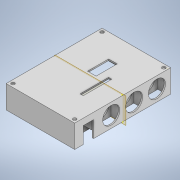
# Autodesk Inventor part: upper casing
Saved by Autodesk Inventor 2020 (Build 240168000, 168)
## iProperties
Created: 2019-06-23
Part Number: upper casing
Material: Generic
Document SubType Name: Modeling
Designer: jjsch
Density: 1 g/cm^3
Appearance: Default
Mass: 122.715 g
Surface Area: 805.458 cm^2
Volume: 122.715 cm^3
Author: jjsch
Autodesk Inventor part; units mm, degrees
ref_plane "YZ Plane" through (0, 0, 0) normal (1, 0, 0) x (0, 1, 0)
ref_plane "XZ Plane" through (0, 0, 0) normal (0, 1, 0) x (-1, 0, 0)
ref_plane "XY Plane" through (0, 0, 0) normal (0, 0, 1) x (1, 0, 0)
sketch "Sketch1" plane through (0, 0, 0) normal (0, 1, 0) x (-1, 0, 0)
  line L0 (-1.2, -80) -> (1.2, -80)
  line L1 (1.2, -80) -> (1.2, 80)
  line L2 (1.2, 80) -> (-1.2, 80)
  line L3 (-1.2, 80) -> (-1.2, -80)
  line L4 (-1.2, -80) -> (1.2, 80) construction
  line L5 (1.2, -80) -> (-1.2, 80) construction
  point P0 (0, 0)
  dimension "d0" = 2.4
  dimension "d1" = 160
  constraints: 12 end point, 2 midpoint, 2 parallel, 1 horizontal, 1 perpendicular
  measures "d0" distance of L2.end L1.end
  measures "d1" distance of L1.end L0.end
extrude "Extrusion1" add sketch "Sketch1" along normal blind 40
sketch "Sketch2" plane through (1.2, 0, 80) normal (1, 0, 0) x (0, 0, -1)
  line L0 (0, 0) -> (0, 40) projected
  line L1 (160, 0) -> (160, 40) projected
  circle A0 centre (60, 20) radius 15
  circle A1 centre (100, 20) radius 15
  circle A2 centre (140, 20) radius 15
  line L2 (29.05, 28.75) -> (10.95, 28.75)
  line L3 (10.95, 28.75) -> (10.95, 11.25)
  line L4 (10.95, 11.25) -> (29.05, 11.25)
  line L5 (29.05, 11.25) -> (29.05, 28.75)
  line L6 (29.05, 28.75) -> (10.95, 11.25) construction
  line L7 (10.95, 28.75) -> (29.05, 11.25) construction
  point P0 (80, 0)
  point P1 (20, 20)
  dimension "d4" = 60
  dimension "d5" = 20
  dimension "d6" = 40
  dimension "d7" = 20
  dimension "d8" = 30
  dimension "d9" = 30
  dimension "d10" = 30
  dimension "d11" = 18.1
  dimension "d12" = 17.5
  constraints: 12 end point, 3 centre point, 3 coincident, 2 midpoint, 2 parallel, 1 horizontal, 1 perpendicular
  measures "d4" distance from line of L0 point (60, 20)
  measures "d5" distance from line of L1 point (140, 20)
  measures "d6" distance of point (140, 20) point (100, 20)
  measures "d7" distance from line of L0 point (20, 20)
  measures "d8" diameter of A0
  measures "d9" diameter of A1
  measures "d10" diameter of A2
  measures "d11" distance of L4.end L3.end
  measures "d12" distance of L3.end L2.end
extrude "Extrusion2" cut sketch "Sketch2" against normal blind 40
sketch "Sketch3" plane through (1.2, 0, -80) normal (0, 0, -1) x (-1, 0, 0)
  line L0 (2.4, 0) -> (2.4, 40) projected
  point P0 (1.2, 0)
sketch "Sketch4" plane through (0, 40, 0) normal (0, 1, 0) x (1, 0, 0)
  line L0 (1.2, -80) -> (-118.8, -80)
  line L1 (-118.8, -80) -> (-118.8, 80)
  line L2 (-118.8, 80) -> (1.2, 80)
  line L3 (1.2, 80) -> (1.2, -80)
  point P0 (0, 0)
  dimension "d17" = 120
  dimension "d18" = 160
  constraints: 8 end point, 2 parallel, 1 horizontal, 1 perpendicular
  measures "d17" distance of L1.end L2.end
  measures "d18" distance of L0.end L1.end
extrude "Extrusion3" add sketch "Sketch4" against normal blind 2.4
sketch "Sketch5" plane through (-1.2, 0, -80) normal (-1, 0, 0) x (0, 0, 1)
  circle A0 centre (20, 20) radius 15 projected
  circle A1 centre (60, 20) radius 15 projected
  circle A2 centre (100, 20) radius 15 projected
  line L0 (160, 37.6) -> (0, 37.6) projected
  line L1 (9, 37.6) -> (31, 37.6)
  line L2 (31, 30.198) -> (31, 37.6)
  line L3 (9, 37.6) -> (9, 30.198)
  arc A3 (31, 30.198) -> (9, 30.198) centre (20, 20) ccw
  arc A4 (71, 30.198) -> (49, 30.198) centre (60, 20) ccw
  arc A5 (111, 30.198) -> (89, 30.198) centre (100, 20) ccw
  line L4 (49, 30.198) -> (49, 37.6)
  line L5 (49, 37.6) -> (71, 37.6)
  line L6 (71, 37.6) -> (71, 30.198)
  line L7 (89, 30.198) -> (89, 37.6)
  line L8 (89, 37.6) -> (111, 37.6)
  line L9 (111, 37.6) -> (111, 30.198)
  point P0 (80, 0)
  constraints: 18 end point, 12 point on circle, 6 point on line, 5 perpendicular, 3 centre point, 3 concentric, 1 parallel
extrude "Extrusion4" add sketch "Sketch5" along normal blind 28.6 contours A0 L3 L0 L2 | A1 L4 L0 L6 | A2 L7 L0 L9
sketch "Sketch6" plane through (-1.2, 0, -80) normal (-1, 0, 0) x (0, 0, 1)
  point P0 (80, 0)
sketch "Sketch7" plane through (-1.2, 0, -80) normal (-1, 0, 0) x (0, 0, 1)
  line L0 (160, 0) -> (160, 37.6) projected
  line L1 (150.3, 30.05) -> (129.7, 30.05)
  line L2 (129.7, 30.05) -> (129.7, 9.95)
  line L3 (129.7, 9.95) -> (150.3, 9.95)
  line L4 (150.3, 9.95) -> (150.3, 30.05)
  line L5 (150.3, 30.05) -> (129.7, 9.95) construction
  line L6 (129.7, 30.05) -> (150.3, 9.95) construction
  line L7 (130.95, 11.25) -> (130.95, 28.75)
  line L8 (149.05, 28.75) -> (149.05, 11.25)
  line L9 (149.05, 11.25) -> (130.95, 28.75) construction
  line L10 (130.95, 11.25) -> (149.05, 28.75) construction
  line L11 (128.5, 8.65) -> (151.5, 8.65)
  line L12 (151.5, 8.65) -> (151.5, 31.35)
  line L13 (151.5, 31.35) -> (128.5, 31.35)
  line L14 (128.5, 31.35) -> (128.5, 8.65)
  line L15 (128.5, 8.65) -> (151.5, 31.35) construction
  line L16 (151.5, 8.65) -> (128.5, 31.35) construction
  point P0 (80, 0)
  point P1 (140, 20)
  dimension "d25" = 20.6
  dimension "d26" = 20.1
  dimension "d27" = 23
  dimension "d28" = 22.7
  constraints: 32 end point, 6 midpoint, 5 parallel, 2 horizontal, 2 perpendicular
  measures "d25" distance of L3.end L2.end
  measures "d26" distance of L2.end L1.end
  measures "d27" distance of L13.end L12.end
  measures "d28" distance of L12.end L11.end
extrude "Extrusion5" add sketch "Sketch7" along normal blind 1.45
sketch "Sketch8" plane through (-2.65, 0, -80) normal (-1, 0, 0) x (0, 0, 1)
  line L0 (149.05, 28.75) -> (149.05, 11.25) projected
  line L1 (130.95, 11.25) -> (149.05, 11.25)
  line L2 (149.05, 11.25) -> (149.05, 28.75)
  line L3 (149.05, 28.75) -> (130.95, 28.75)
  line L4 (130.95, 28.75) -> (130.95, 11.25)
  line L5 (130.95, 11.25) -> (149.05, 28.75) construction
  line L6 (149.05, 11.25) -> (130.95, 28.75) construction
  line L7 (128.5, 31.35) -> (128.5, 8.65) projected
  line L8 (151.5, 8.65) -> (128.5, 8.65)
  line L9 (128.5, 8.65) -> (128.5, 31.35)
  line L10 (128.5, 31.35) -> (151.5, 31.35)
  line L11 (151.5, 31.35) -> (151.5, 8.65)
  line L12 (151.5, 8.65) -> (128.5, 31.35) construction
  line L13 (128.5, 8.65) -> (151.5, 31.35) construction
  point P0 (80, 0)
  point P1 (140, 20)
  constraints: 24 end point, 4 midpoint, 4 parallel, 2 horizontal, 2 perpendicular
extrude "Extrusion6" add sketch "Sketch8" along normal blind 19.65
sketch "Sketch9" plane through (-22.3, 0, -80) normal (-1, 0, 0) x (0, 0, 1)
  line L0 (149.05, 11.25) -> (130.95, 11.25) projected
  line L1 (149.05, 11.25) -> (123.685, 11.25)
  line L2 (123.685, 11.25) -> (123.685, 3.7797)
  line L3 (123.685, 3.7797) -> (156.7839, 3.4557)
  line L4 (156.7839, 3.4557) -> (156.8602, 11.25)
  line L5 (156.8602, 11.25) -> (149.3348, 11.25)
  line L6 (149.05, 28.75) -> (149.05, 11.25) projected
  line L7 (149.3348, 11.25) -> (149.05, 11.25)
  point P0 (80, 0)
  constraints: 12 end point, 2 perpendicular, 2 point on line, 1 collinear, 1 horizontal
extrude "Extrusion7" cut sketch "Sketch9" against normal up to surface (21.1 mm away)
sketch "Sketch10" plane through (1.2, 0, 80) normal (1, 0, 0) x (0, 0, -1)
  line L0 (10.95, 11.25) -> (29.05, 11.25) projected
  line L1 (10.95, 11.25) -> (29.05, 11.25)
  line L2 (29.05, 11.25) -> (29.05, -6.8094)
  line L3 (29.05, -6.8094) -> (10.95, -6.8094)
  line L4 (10.95, -6.8094) -> (10.95, 11.25)
  point P0 (80, 0)
  constraints: 8 end point, 2 parallel, 1 horizontal, 1 perpendicular
extrude "Extrusion8" cut sketch "Sketch10" against normal blind 19.65
sketch "Sketch11" plane through (-1.2, 0, -80) normal (-1, 0, 0) x (0, 0, 1)
  line L0 (128.5, 31.35) -> (128.5, 11.25) projected
  line L1 (160, 37.6) -> (111, 37.6) projected
  line L2 (128.5, 31.35) -> (130.95, 31.35)
  line L3 (130.95, 31.35) -> (130.95, 37.6)
  line L4 (130.95, 37.6) -> (128.5, 37.6)
  line L5 (128.5, 37.6) -> (128.5, 31.35)
  line L6 (128.5, 31.35) -> (151.5, 31.35) projected
  line L7 (151.5, 31.35) -> (149.05, 31.35)
  line L8 (149.05, 31.35) -> (149.05, 37.6)
  line L9 (149.05, 37.6) -> (151.5, 37.6)
  line L10 (151.5, 37.6) -> (151.5, 31.35)
  line L11 (141.225, 31.35) -> (138.775, 31.35)
  line L12 (138.775, 31.35) -> (138.775, 37.6)
  line L13 (138.775, 37.6) -> (141.225, 37.6)
  line L14 (141.225, 37.6) -> (141.225, 31.35)
  line L15 (141.225, 31.35) -> (138.775, 37.6) construction
  line L16 (138.775, 31.35) -> (141.225, 37.6) construction
  line L17 (130.95, 37.6) -> (138.775, 31.35)
  line L18 (130.95, 36.3) -> (137.1474, 31.35)
  line L19 (137.1474, 31.35) -> (138.775, 31.35)
  line L20 (138.775, 31.35) -> (138.775, 32.65)
  line L21 (138.775, 32.65) -> (132.5776, 37.6)
  line L22 (132.5776, 37.6) -> (130.95, 37.6)
  line L23 (130.95, 37.6) -> (130.95, 36.3)
  line L24 (140, 34.475) -> (140, 37.6)
  line L25 (149.05, 37.6) -> (141.225, 31.35)
  line L26 (149.05, 36.3) -> (142.8526, 31.35)
  line L27 (141.225, 32.65) -> (147.4224, 37.6)
  line L28 (147.4224, 37.6) -> (149.05, 37.6)
  line L29 (149.05, 37.6) -> (149.05, 36.3)
  line L30 (142.8526, 31.35) -> (141.225, 31.35)
  line L31 (138.775, 31.35) -> (137.1474, 31.35)
  line L32 (130.95, 36.3) -> (130.95, 37.6)
  point P0 (80, 0)
  dimension "d37" = 2.45
  dimension "d38" = 2.45
  dimension "d39" = 2.45
  dimension "d40" = 1.3
  constraints: 60 end point, 8 parallel, 8 point on line, 5 collinear, 5 perpendicular, 4 symmetric about line, 3 horizontal, 3 midpoint
  measures "d37" distance of L4.end L3.end
  measures "d38" distance of L8.end L9.end
  measures "d39" distance of L12.end L13.end
  measures "d40" distance of L11.end L20.end
extrude "Extrusion9" add sketch "Sketch11" along normal up to surface (21.1 mm away) contours L10 L6 L8 L1 | L25 L14 L27 L1 | L8 L26 L6 L25 | L6 L12 L1 L14 | L17 L1 L21 L12 | L6 L18 L3 L17 | L3 L2 L5 L1
sketch "Sketch12" plane through (1.2, 0, -80) normal (0, 0, -1) x (-1, 0, 0)
  line L0 (0, 40) -> (120, 40) projected
  line L1 (0, 40) -> (120, 40)
  line L2 (120, 40) -> (120, 0)
  line L3 (120, 0) -> (0, 0)
  line L4 (0, 0) -> (0, 40)
  point P0 (1.2, 0)
  dimension "d96" = 120
  constraints: 8 end point, 2 parallel, 1 horizontal, 1 perpendicular
  measures "d96" distance of L2.end L3.end
extrude "Extrusion10" add sketch "Sketch12" along normal blind 4
sketch "Sketch13" plane through (0, 37.6, 0) normal (0, -1, 0) x (1, 0, 0)
  point P0 (0, 0)
sketch "Sketch14" plane through (1.2, 0, 80) normal (0, 0, 1) x (1, 0, 0)
  line L0 (-120, 40) -> (-120, 37.6) projected
  line L1 (-2.4, 0) -> (0, 0) projected
  line L2 (-120, 40) -> (0, 40)
  line L3 (0, 40) -> (0, 0)
  line L4 (0, 0) -> (-120, 0)
  line L5 (-120, 0) -> (-120, 40)
  point P0 (-1.2, 0)
  constraints: 8 end point, 2 parallel, 1 horizontal, 1 perpendicular
extrude "Extrusion11" add sketch "Sketch14" along normal blind 4
sketch "Sketch15" plane through (1.2, 0, 69.05) normal (1, 0, 0) x (0, 0, -1)
  point P0 (69.05, 0)
sketch "Sketch16" plane through (0, 37.6, 0) normal (0, -1, 0) x (1, 0, 0)
  line L0 (-1.2, 80) -> (-118.8, 80) projected
  line L1 (-22.3, 80) -> (-17.3, 80)
  line L2 (-17.3, 80) -> (-17.3, -80)
  line L3 (-17.3, -80) -> (-22.3, -80)
  line L4 (-22.3, -80) -> (-22.3, 80)
  point P0 (0, 0)
  dimension "d47" = 5
  dimension "d48" = 160
  constraints: 8 end point, 2 parallel, 1 horizontal, 1 perpendicular, 1 point on line
  measures "d47" distance of L2.end L3.end
  measures "d48" distance of L1.end L2.end
extrude "Extrusion12" add sketch "Sketch16" along normal up to surface (37.6 mm away)
sketch "Sketch17" plane through (1.2, 0, 69.05) normal (1, 0, 0) x (0, 0, -1)
  line L0 (0, 28.75) -> (18.1, 28.75) projected
  line L1 (0, 28.75) -> (18.1, 28.75)
  line L2 (18.1, 28.75) -> (18.1, 0)
  line L3 (18.1, 0) -> (0, 0)
  line L4 (0, 0) -> (0, 28.75)
  point P0 (69.05, 0)
  constraints: 8 end point, 2 parallel, 1 horizontal, 1 perpendicular
extrude "Extrusion13" cut sketch "Sketch17" against normal blind 4000
sketch "Sketch18" plane through (1.2, 0, 69.05) normal (1, 0, 0) x (0, 0, -1)
  point P0 (69.05, 0)
sketch "Sketch19" plane through (-17.3, 37.6, -31) normal (1, 0, 0) x (0, 0, -1)
  arc A0 (-62, -7.402) -> (-40, -7.402) centre (-51, -17.6) ccw projected
  circle A1 centre (-51, -17.6) radius 15
  arc A2 (0, -7.402) -> (-22, -7.402) centre (-11, -17.6) ccw projected
  circle A3 centre (-11, -17.6) radius 15
  arc A4 (40, -7.402) -> (18, -7.402) centre (29, -17.6) ccw projected
  circle A5 centre (29, -17.6) radius 15
  point P0 (-31, -37.6)
  point P1 (18, -7.402)
  point P2 (40, -7.402)
  point P3 (-22, -7.402)
  point P4 (0, -7.402)
  point P5 (-40, -7.402)
  point P6 (-62, -7.402)
  constraints: 3 centre point, 3 coincident
extrude "Extrusion14" cut sketch "Sketch19" against normal blind 4000
sketch "Sketch20" plane through (0, 37.6, 0) normal (0, -1, 0) x (1, 0, 0)
  line L0 (-1.2, -80) -> (-1.2, 50.95) projected
  line L1 (-1.2, 0) -> (-22.3, 0)
  line L2 (-22.3, 50.95) -> (-22.3, -80) projected
  line L3 (-22.3, 0) -> (-22.3, -2)
  line L4 (-22.3, -2) -> (-1.2, -2)
  line L5 (-1.2, -2) -> (-1.2, 0)
  line L6 (-1.2, 0) -> (-1.2, 2)
  line L7 (-1.2, 2) -> (-22.3, 2)
  line L8 (-22.3, 2) -> (-22.3, 0)
  point P0 (0, 0)
  dimension "d55" = 2
  dimension "d56" = 2
  constraints: 14 end point, 4 perpendicular, 4 point on line, 1 collinear, 1 horizontal
  measures "d55" distance of L1.end L3.end
  measures "d56" distance of L1.start L6.end
extrude "Extrusion15" add sketch "Sketch20" along normal up to surface (37.6 mm away)
sketch "Sketch21" plane through (0, 37.6, 0) normal (0, -1, 0) x (1, 0, 0)
  line L0 (-1.2, -80) -> (-1.2, -2) projected
  line L1 (-17.3, -80) -> (-17.3, -2) projected
  line L2 (-1.2, -49) -> (-17.3, -49) projected
  line L3 (-1.2, -31) -> (-17.3, -31) projected
  line L4 (-17.3, -38) -> (-1.2, -38)
  line L5 (-1.2, -38) -> (-1.2, -42)
  line L6 (-1.2, -42) -> (-17.3, -42)
  line L7 (-17.3, -42) -> (-17.3, -38)
  line L8 (-17.3, -38) -> (-1.2, -42) construction
  line L9 (-1.2, -38) -> (-17.3, -42) construction
  point P0 (0, 0)
  point P1 (-9.25, -40)
  point P2 (-1.2, -38)
  dimension "d59" = 8.05
  dimension "d60" = 8.05
  dimension "d61" = 9
  dimension "d62" = 9
  dimension "d63" = 16.1
  dimension "d64" = 4
  constraints: 12 end point, 2 midpoint, 2 parallel, 1 horizontal, 1 perpendicular
  measures "d59" distance from line of L0 point (-9.25, -40)
  measures "d60" distance from line of L1 point (-9.25, -40)
  measures "d61" distance from line of L2 point (-9.25, -40)
  measures "d62" distance from line of L3 point (-9.25, -40)
  measures "d63" distance of L5.end L6.end
  measures "d64" distance of L4.end L5.end
extrude "Extrusion16" add sketch "Sketch21" along normal up to surface (37.6 mm away) contours L6 L1 L4 L0
sketch "Sketch22" plane through (0, 37.6, 0) normal (0, -1, 0) x (1, 0, 0)
  point P0 (0, 0)
sketch "Sketch23" plane through (0, 37.6, 0) normal (0, -1, 0) x (1, 0, 0)
  line L0 (-118.8, 80) -> (-118.8, -80) projected
  line L1 (-22.3, 80) -> (-118.8, 80) projected
  circle A0 centre (-66.3, 76.5) radius 3
  circle A1 centre (-115.3, 76.5) radius 3
  circle A2 centre (-115.3, 18.5) radius 3
  circle A3 centre (-66.3, 18.5) radius 3
  circle A4 centre (-66.3, 18.5) radius 1.375
  circle A5 centre (-115.3, 18.5) radius 1.375
  circle A6 centre (-115.3, 76.5) radius 1.375
  circle A7 centre (-66.3, 76.5) radius 1.375
  point P0 (0, 0)
  dimension "d67" = 58
  dimension "d68" = 58
  dimension "d69" = 49
  dimension "d70" = 3.5
  dimension "d71" = 3.5
  dimension "d72" = 6
  dimension "d73" = 6
  dimension "d74" = 6
  dimension "d75" = 6
  dimension "d78" = 2.75
  dimension "d79" = 2.75
  dimension "d80" = 2.75
  dimension "d81" = 2.75
  constraints: 8 centre point, 8 coincident, 2 vertical alignment, 1 horizontal alignment
  measures "d67" distance of point (-66.3, 18.5) point (-66.3, 76.5)
  measures "d68" distance of point (-115.3, 18.5) point (-115.3, 76.5)
  measures "d69" distance of point (-66.3, 18.5) point (-115.3, 18.5)
  measures "d70" distance from line of L0 point (-115.3, 76.5)
  measures "d71" distance from line of L1 point (-115.3, 76.5)
  measures "d72" diameter of A0
  measures "d73" diameter of A1
  measures "d74" diameter of A2
  measures "d75" diameter of A3
  measures "d78" diameter of A4
  measures "d79" diameter of A5
  measures "d80" diameter of A6
  measures "d81" diameter of A7
extrude "Extrusion17" add sketch "Sketch23" along normal blind 8
ref_plane "Work Plane1" through (-1.2, 0, 0) normal (0, 0, 1) x (1, 0, 0)
sketch "Sketch28" plane through (0, 0, 0) normal (0, -1, 0) x (1, 0, 0)
  point P0 (0, 0)
sketch "Sketch29" plane through (0, 37.6, 0) normal (0, -1, 0) x (1, 0, 0)
  circle A0 centre (-115.3, 18.5) radius 3 projected
  circle A1 centre (-66.3, 18.5) radius 3 projected
  circle A2 centre (-115.3, 76.5) radius 3 projected
  circle A3 centre (-66.3, 76.5) radius 3 projected
  line L0 (-22.3, -80) -> (-22.3, -71) projected
  line L1 (-22.3, -71) -> (-29.8, -71) projected
  line L2 (-29.8, -71) -> (-29.8, -49) projected
  line L3 (-29.8, -49) -> (-22.3, -49) projected
  line L4 (-22.3, -49) -> (-22.3, -31) projected
  line L5 (-22.3, -31) -> (-29.8, -31) projected
  line L6 (-29.8, -31) -> (-29.8, -9) projected
  line L7 (-29.8, -9) -> (-22.3, -9) projected
  line L8 (-22.3, -9) -> (-22.3, 9) projected
  line L9 (-22.3, 9) -> (-29.8, 9) projected
  line L10 (-29.8, 9) -> (-29.8, 31) projected
  line L11 (-29.8, 31) -> (-22.3, 31) projected
  line L12 (-22.3, 31) -> (-22.3, 80) projected
  line L13 (-22.3, 80) -> (-118.8, 80) projected
  line L14 (-118.8, 80) -> (-118.8, -80) projected
  line L15 (-118.8, -80) -> (-22.3, -80) projected
  line L16 (-35.8, -3) -> (-35.8, -37)
  line L17 (-35.8, -37) -> (-28.3, -37)
  line L18 (-28.3, -37) -> (-28.3, -43)
  line L19 (-28.3, -43) -> (-35.8, -43)
  line L20 (-35.8, -43) -> (-35.8, -74)
  line L21 (-35.8, -74) -> (-112.8, -74)
  line L22 (-112.8, -74) -> (-112.8, 74)
  line L23 (-112.8, 74) -> (-28.3, 74)
  line L24 (-28.3, 74) -> (-28.3, 37)
  line L25 (-28.3, 37) -> (-35.8, 37)
  line L26 (-35.8, 37) -> (-35.8, 3)
  line L27 (-35.8, 3) -> (-28.3, 3)
  line L28 (-28.3, 3) -> (-28.3, -3)
  line L29 (-28.3, -3) -> (-35.8, -3)
  line L30 (-112.8, -74) -> (-35.8, -74)
  line L31 (-35.8, -74) -> (-35.8, -6)
  line L32 (-35.8, -6) -> (-112.8, -6)
  line L33 (-112.8, -6) -> (-112.8, -74)
  line L34 (-66.3, -74) -> (-51.3, -74)
  line L35 (-51.3, -74) -> (-51.3, -6)
  line L36 (-51.3, -6) -> (-66.3, -6)
  line L37 (-66.3, -6) -> (-66.3, -74)
  line L38 (-51.3, -51.2056) -> (-36.3, -51.2056) construction
  line L39 (-118.8, -84) -> (1.2, -84) projected
  line L40 (-59.1553, -43) -> (-66.3, -43)
  line L41 (-59.1553, -43) -> (-51.3, -43)
  line L42 (-142.8, 0) -> (25.2, 0) projected
  point P0 (0, 0)
  point P1 (-66.3, -6)
  dimension "d97" = 6
  dimension "d98" = 15
  dimension "d110" = 41
  dimension "d118" = 6
  constraints: 50 end point, 6 point on line, 4 parallel, 3 horizontal, 3 perpendicular, 13 other
  measures "d97" distance between parallel lines of L6 L16
  measures "d98" distance of L36.end L35.end
  measures "d110" distance from line of L39 L40.start
  measures "d118" distance between parallel lines of L42 L32
extrude "Extrusion20" cut sketch "Sketch29" along normal mid plane 10 contours L32 L35 L41 L40 L37
sketch "Sketch30" plane through (0, 40, 0) normal (0, 1, 0) x (1, 0, 0)
  line L0 (-51.3, 43) -> (-51.3, 6) projected
  line L1 (-51.3, 6) -> (-66.3, 6) projected
  line L2 (-66.3, 6) -> (-66.3, 43) projected
  line L3 (1.2, 84) -> (1.2, -84) projected
  line L4 (-118.8, 84) -> (1.2, 84) projected
  line L5 (-118.8, 84) -> (-118.8, -84) projected
  line L6 (1.2, -84) -> (-118.8, -84) projected
  line L7 (-112.8, -78) -> (-112.8, 78)
  line L8 (-112.8, 78) -> (-4.8, 78)
  line L9 (-4.8, 78) -> (-4.8, -78)
  line L10 (-4.8, -78) -> (-112.8, -78)
  circle A0 centre (-112.8, -78) radius 3
  circle A1 centre (-112.8, 78) radius 3
  circle A2 centre (-4.8, -78) radius 3
  circle A3 centre (-4.8, 78) radius 3
  line L11 (-66.3, 43) -> (-51.3, 43) projected
  point P0 (0, 0)
  dimension "d101" = 6
  dimension "d102" = 6
  dimension "d103" = 6
  dimension "d104" = 6
  dimension "d105" = 6
  constraints: 8 coincident, 8 end point, 4 centre point, 3 other
  measures "d101" distance between parallel lines of L6 L10
  measures "d102" diameter of A0
  measures "d103" diameter of A1
  measures "d104" diameter of A2
  measures "d105" diameter of A3
sketch "Sketch31" plane through (0, 40, 0) normal (0, 1, 0) x (1, 0, 0)
  point P0 (0, 0)
extrude "Extrusion21" cut sketch "Sketch30" against normal blind 2 contours L10 A0 L7 | L7 A0 L10 | A1 L8 L7 | L7 L8 A1 | A2 L9 L10 | L10 L9 A2 | A3 L9 L8 | L8 L9 A3
sketch "Sketch32" plane through (0, 40, 0) normal (0, 1, 0) x (1, 0, 0)
  line L0 (1.2, 84) -> (1.2, -84) projected
  line L1 (-118.8, 84) -> (1.2, 84) projected
  line L2 (-32.842, -35) -> (-32.842, 15)
  line L3 (-32.842, 15) -> (-38.382, 15)
  line L4 (-38.382, 15) -> (-38.382, -35)
  line L5 (-38.382, -35) -> (-32.842, -35)
  point P0 (0, 0)
  dimension "d111" = 50
  dimension "d112" = 34.042
  dimension "d113" = 34.042
  dimension "d114" = 69
  dimension "d115" = 5.54
  constraints: 8 end point, 3 perpendicular
  measures "d111" distance of L2.end L2.start
  measures "d112" distance from line of L0 L2.start
  measures "d113" distance from line of L0 L2.end
  measures "d114" distance from line of L1 L2.end
  measures "d115" distance of L2.end L3.end
extrude "Extrusion22" cut sketch "Sketch32" against normal blind 10
sketch "Sketch33" plane through (0, 37.6, 0) normal (0, -1, 0) x (1, 0, 0)
  point P0 (0, 0)
sketch "Sketch34" plane through (0, 40, 0) normal (0, 1, 0) x (1, 0, 0)
  point P0 (0, 0)
body "Solid1"
